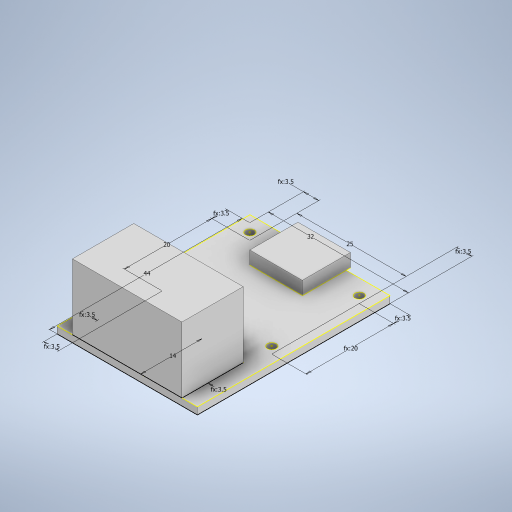
# Autodesk Inventor part: MOSFET_Controller
Saved by Autodesk Inventor 2024 (Build 280153000, 153)
## iProperties
Created: 2025-11-07
Part Number: MOSFET_Controller
Material: 일반
Document SubType Name: Modeling
Designer: alexi
Density: 1 g/cm^3
Appearance: 기본값
Author: alexi
Autodesk Inventor part; units mm, degrees
ref_plane "YZ Plane" through (0, 0, 0) normal (1, 0, 0) x (0, 1, 0)
ref_plane "XZ Plane" through (0, 0, 0) normal (0, 1, 0) x (-1, 0, 0)
ref_plane "XY Plane" through (0, 0, 0) normal (0, 0, 1) x (1, 0, 0)
sketch "스케치1" plane through (0, 0, 0) normal (0, 1, 0) x (-1, 0, 0)
  line L0 (16, 22) -> (-16, 22)
  line L1 (-16, 22) -> (-16, -22)
  line L2 (-16, -22) -> (16, -22)
  line L3 (16, -22) -> (16, 22)
  line L4 (-16, 22) -> (16, -22) construction
  line L5 (16, 22) -> (-16, -22) construction
  point P0 (0, 0)
  point P1 (0, 0)
  point P2 (12.5, -18.5)
  point P3 (12.5, 1.5)
  point P4 (-12.5, 1.5)
  point P5 (-12.5, -18.5)
  dimension "d0" = 44
  dimension "d1" = 32
  dimension "d2" = 25
  dimension "d3" = 3.5
  dimension "d4" = 3.5
  dimension "d5" = 3.5
  dimension "d6" = 20
  dimension "d7" = 20
  dimension "d8" = 3.5
  dimension "d9" = 3.5
  constraints: 12 end point, 2 midpoint, 2 parallel, 1 coincident, 1 horizontal, 1 perpendicular
  measures "d0" distance of L2.end L0.start
  measures "d1" distance of L1.end L2.end
  measures "d2" distance of point (12.5, -18.5) point (-12.5, -18.5)
  measures "d3" distance from line of L3 point (12.5, -18.5)
  measures "d4" distance from line of L2 point (12.5, -18.5)
  measures "d5" distance from line of L2 point (-12.5, -18.5)
  measures "d6" distance of point (12.5, -18.5) point (12.5, 1.5)
  measures "d7" distance of point (-12.5, -18.5) point (-12.5, 1.5)
  measures "d8" distance from line of L3 point (12.5, 1.5)
  measures "d9" distance from line of L1 point (-12.5, 1.5)
extrude "돌출1" add sketch "스케치1" along normal blind 1.6
hole "구멍1" at (-12.5, 0, 1.5) at (-12.5, 0, -18.5) at (12.5, 0, -18.5) at (12.5, 0, 1.5) direction (0, 1, 0) diameter 2 depth 1.6
sketch "스케치2" plane through (0, 1.6, 0) normal (0, 1, 0) x (1, 0, 0)
  line L0 (-16, -22) -> (16, -22) projected
  line L1 (-12.5, -22) -> (12.5, -22)
  line L2 (12.5, -22) -> (12.5, -8)
  line L3 (12.5, -8) -> (-12.5, -8)
  line L4 (-12.5, -8) -> (-12.5, -22)
  line L5 (-16, 22) -> (-16, -22) projected
  line L6 (16, -22) -> (16, 22) projected
  point P0 (0, 0)
  dimension "d19" = 3.5
  dimension "d20" = 3.5
  dimension "d21" = 14
  constraints: 8 end point, 2 parallel, 1 horizontal, 1 perpendicular, 1 point on line
  measures "d19" distance between parallel lines of L5 L4
  measures "d20" distance between parallel lines of L6 L2
  measures "d21" distance between parallel lines of L0 L3
extrude "돌출2" add sketch "스케치2" along normal blind 15
sketch "스케치3" plane through (0, 1.6, 0) normal (0, 1, 0) x (1, 0, 0)
  line L0 (-6, 23) -> (6, 23)
  line L1 (6, 23) -> (6, 12)
  line L2 (6, 12) -> (-6, 12)
  line L3 (-6, 12) -> (-6, 23)
  line L4 (16, 22) -> (-16, 22) projected
  point P0 (0, 0)
  dimension "d24" = 10
  dimension "d25" = 6
  dimension "d26" = 6
  dimension "d27" = 1
  constraints: 8 end point, 2 parallel, 1 horizontal, 1 perpendicular
  measures "d24" distance between parallel lines of L2 L4
  measures "d25" distance from line of point (0, 0) L3
  measures "d26" distance from line of point (0, 0) L1
  measures "d27" distance between parallel lines of L4 L0
extrude "돌출3" add sketch "스케치3" along normal blind 3
sketch "스케치4" plane through (0, 1.6, 0) normal (0, 1, 0) x (1, 0, 0)
  line L0 (-6, 12) -> (-6, 22) projected
  line L1 (-6, 22) -> (-16, 22) projected
  line L2 (-16, 22) -> (-16, -22) projected
  line L3 (-16, -22) -> (-12.5, -22) projected
  line L4 (-12.5, -22) -> (-12.5, -8) projected
  line L5 (-12.5, -8) -> (12.5, -8) projected
  line L6 (12.5, -8) -> (12.5, -22) projected
  line L7 (12.5, -22) -> (16, -22) projected
  line L8 (16, -22) -> (16, 22) projected
  line L9 (16, 22) -> (6, 22) projected
  line L10 (6, 22) -> (6, 12) projected
  line L11 (6, 12) -> (-6, 12) projected
  circle A0 centre (12.5, -1.5) radius 1 projected
  circle A1 centre (12.5, 18.5) radius 1 projected
  circle A2 centre (-12.5, 18.5) radius 1 projected
  circle A3 centre (-12.5, -1.5) radius 1 projected
  line L12 (6, 12) -> (6, 23) projected
  line L13 (6, 23) -> (-6, 23) projected
  line L14 (-6, 23) -> (-6, 12) projected
  line L15 (-6, 12) -> (6, 12) projected
  line L16 (-12.5, -8) -> (-12.5, -22) projected
  line L17 (-12.5, -22) -> (12.5, -22) projected
  line L18 (12.5, -22) -> (12.5, -8) projected
  line L19 (12.5, -8) -> (-12.5, -8) projected
  point P0 (0, 0)
equation "\"d3\" = -0.5 * d2 + 0.5 * d1"
equation "\"d4\" = d3"
equation "\"d5\" = d4"
equation "\"d7\" = d6"
equation "\"d8\" = d3"
equation "\"d9\" = d3"
equation "\"d19\" = d3"
equation "\"d20\" = d9"
equation "\"d26\" = d25"
